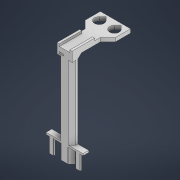
# Autodesk Inventor part: Vertical Beam Prototype
Saved by Autodesk Inventor 2022 (Build 260153000, 153)
## iProperties
Created: 2021-05-30
Part Number: Vertical Beam Prototype
Material: Generic
Document SubType Name: Modeling
Designer: sidsa
Density: 1 g/cm^3
Appearance: Default
Author: sidsa
## iProperties of the stored document Vertical Beam Prototype_3DPrint.ipt
Created: 2021-05-30
Part Number: Vertical Beam Prototype_3DPrint
Material: Generic
Document SubType Name: Modeling
Designer: sidsa
Density: 1 g/cm^3
Appearance: Default
Author: sidsa
Autodesk Inventor part; units mm, degrees
ref_plane "YZ Plane" through (0, 0, 0) normal (1, 0, 0) x (0, 1, 0)
ref_plane "XZ Plane" through (0, 0, 0) normal (0, 1, 0) x (-1, 0, 0)
ref_plane "XY Plane" through (0, 0, 0) normal (0, 0, 1) x (1, 0, 0)
sketch "Sketch1" plane through (0, 0, 0) normal (0, 0, 1) x (1, 0, 0)
  line L0 (0, 0) -> (25.4, 0)
  line L1 (25.4, 0) -> (25.4, 165.1)
  line L2 (25.4, 165.1) -> (0, 165.1)
  line L3 (0, 165.1) -> (0, 0)
  line L4 (16.2837, 38.7604) -> (19.9133, 32.4739)
  line L5 (19.9133, 32.4739) -> (16.2837, 26.1874)
  line L6 (16.2837, 26.1874) -> (9.0247, 26.1874)
  line L7 (9.0247, 26.1874) -> (5.3952, 32.4739)
  line L8 (5.3952, 32.4739) -> (9.0247, 38.7604)
  line L9 (9.0247, 38.7604) -> (16.2837, 38.7604)
  line L10 (12.7, 0) -> (12.6542, 32.4739)
  dimension "d0" = 25.4
  dimension "d1" = 165.1
  dimension "d2" = 12.573
  dimension "d3" = 26.1874
  constraints: 22 end point, 3 parallel, 1 horizontal, 1 midpoint, 1 perpendicular, 13 other
  measures "d0" distance of L1.end L2.end
  measures "d1" distance of L0.end L1.end
  measures "d2" distance between parallel lines of L6 L9
  measures "d3" distance between parallel lines of L0 L6
extrude "Extrusion1" add sketch "Sketch1" along normal blind 3.175
sketch "Sketch2" plane through (0, 0, 0) normal (0, 0, -1) x (-1, 0, 0)
  line L0 (-25.4, 0) -> (-25.4, 165.1) projected
  line L1 (0, 0) -> (-25.4, 0) projected
  line L2 (0, 165.1) -> (0, 0) projected
  line L3 (-25.4, 165.1) -> (0, 165.1) projected
  line L4 (-16.2837, 26.1874) -> (-9.0247, 26.1874) projected
  line L5 (-19.9133, 32.4739) -> (-16.2837, 26.1874) projected
  line L6 (-16.2837, 38.7604) -> (-19.9133, 32.4739) projected
  line L7 (-9.0247, 38.7604) -> (-16.2837, 38.7604) projected
  line L8 (-5.3952, 32.4739) -> (-9.0247, 38.7604) projected
  line L9 (-9.0247, 26.1874) -> (-5.3952, 32.4739) projected
  line L10 (-16.2984, 26.1967) -> (-19.9179, 32.4658) projected
  line L11 (-5.4399, 32.4658) -> (-9.0594, 26.1967) projected
  line L12 (-9.0594, 26.1967) -> (-16.2984, 26.1967) projected
  line L13 (-16.2984, 26.1967) -> (-19.9179, 32.4658) projected
  line L14 (-19.9179, 32.4658) -> (-16.2984, 38.735) projected
  line L15 (-16.2984, 38.735) -> (-9.0594, 38.735) projected
  line L16 (-9.0594, 38.735) -> (-5.4399, 32.4658) projected
  line L17 (-41.2539, 1.27) -> (-34.9039, 1.27) projected
  line L18 (15.8961, 1.27) -> (15.8961, 63.5) projected
  line L19 (-41.2539, 63.5) -> (15.8961, 63.5) projected
  line L20 (-41.2539, 1.27) -> (-41.2539, 63.5) projected
  line L21 (6.3711, 1.27) -> (6.3711, 26.67) projected
  line L22 (6.3711, 26.67) -> (9.5461, 26.67) projected
  line L23 (9.5461, 26.67) -> (9.5461, 1.27) projected
  line L24 (9.5461, 1.27) -> (15.8961, 1.27) projected
  line L25 (-34.9039, 1.27) -> (-34.9039, 26.67) projected
  line L26 (-34.9039, 26.67) -> (-31.7289, 26.67) projected
  line L27 (-31.7289, 26.67) -> (-31.7289, 1.27) projected
  line L28 (-31.7289, 1.27) -> (6.3711, 1.27) projected
  dimension "d32" = 12.573
  dimension "d33" = 12.5383
  measures "d32" distance between parallel lines of L7 L4
  measures "d33" distance between parallel lines of L12 L15
extrude "Extrusion2" add sketch "Sketch2" along normal blind 6.35 and the other way blind 3.175 contours L5 L12 L11 L16 L15 L6 L7 L8 L9 L4 | L5 L6 L15 L16 L11 L12
sketch "Sketch3" plane through (0, 0, 3.175) normal (0, 0, 1) x (1, 0, 0)
  line L0 (25.4, 0) -> (25.4, 165.1) projected
  line L1 (25.4, 165.1) -> (0, 165.1) projected
  line L2 (0, 165.1) -> (0, 0) projected
  line L3 (0, 0) -> (25.4, 0) projected
extrude "Extrusion3" add sketch "Sketch3" along normal blind 6.35
chamfer "Chamfer1" distance 6.35 angle 45 2 edges at (25.4, 82.55, 9.525) (0, 82.55, 9.525)
sketch "Sketch5" plane through (9.0247, 38.7604, 0) normal (0, 1, 0) x (1, 0, 0)
  line L0 (7.259, 0) -> (7.259, 6.35) projected
  line L1 (32.2292, 2.54) -> (-24.9208, 2.54) projected
  line L2 (0, 0) -> (0, 6.35) projected
  line L3 (7.259, 0) -> (7.259, 6.35) projected
  line L4 (0, 6.35) -> (0, 0) projected
  line L5 (7.259, 2.54) -> (0, 2.54)
  line L6 (0, 2.54) -> (0, 6.35)
  line L7 (0, 6.35) -> (7.259, 6.35)
  line L8 (7.259, 6.35) -> (7.259, 2.54)
  line L9 (5.989, 3.175) -> (1.27, 3.175)
  line L10 (1.27, 3.175) -> (1.27, 5.715)
  line L11 (1.27, 5.715) -> (5.989, 5.715)
  line L12 (5.989, 5.715) -> (5.989, 3.175)
  point P0 (-9.0247, 0)
  dimension "d25" = 0.635
  dimension "d26" = 1.27
  dimension "d27" = 0.635
  dimension "d28" = 1.27
  dimension "d29" = 2.54
  constraints: 16 end point, 4 parallel, 2 horizontal, 2 perpendicular, 2 point on line
  measures "d25" distance between parallel lines of L1 L9
  measures "d26" distance between parallel lines of L2 L10
  measures "d27" distance between parallel lines of L7 L11
  measures "d28" distance between parallel lines of L0 L12
  measures "d29" distance between parallel lines of L11 L9
extrude "Extrusion5" cut sketch "Sketch5" against normal blind 12.7 contours L9 L10 L11 L12
sketch "Sketch6" plane through (0, 0, 0) normal (0, 0, -1) x (-1, 0, 0)
  line L0 (-25.4, 0) -> (-25.4, 165.1) projected
  line L1 (0, 0) -> (-25.4, 0) projected
  line L2 (0, 165.1) -> (0, 0) projected
  line L3 (-25.4, 165.1) -> (0, 165.1) projected
  line L4 (-16.2837, 26.1874) -> (-9.0247, 26.1874) projected
  line L5 (-19.9133, 32.4739) -> (-16.2837, 26.1874) projected
  line L6 (-16.2837, 38.7604) -> (-19.9133, 32.4739) projected
  line L7 (-9.0247, 38.7604) -> (-16.2837, 38.7604) projected
  line L8 (-5.3952, 32.4739) -> (-9.0247, 38.7604) projected
  line L9 (-9.0247, 26.1874) -> (-5.3952, 32.4739) projected
  line L10 (0, 165.1) -> (0, 0) projected
  line L11 (-25.4, 165.1) -> (0, 165.1)
  line L12 (0, 165.1) -> (0, 158.75)
  line L13 (0, 158.75) -> (-25.4, 158.75)
  line L14 (-25.4, 158.75) -> (-25.4, 165.1)
  point P0 (-25.4, 158.75)
  dimension "d34" = 6.35
  constraints: 8 end point, 2 parallel, 1 horizontal, 1 perpendicular, 1 point on line
  measures "d34" distance of L11.end L12.end
extrude "Extrusion6" add sketch "Sketch6" along normal blind 76.2 contours L0 L3 L2 L13
sketch "Sketch7" plane through (0, 0, 3.175) normal (-1, 0, 0) x (0, 0, 1)
  line L0 (-79.375, 165.1) -> (0, 165.1) projected
  line L1 (-3.175, 158.75) -> (-79.375, 158.75) projected
  line L2 (-79.375, 165.1) -> (-53.975, 165.1)
  line L3 (-53.975, 165.1) -> (-53.975, 158.75)
  line L4 (-53.975, 158.75) -> (-79.375, 158.75)
  line L5 (-79.375, 158.75) -> (-79.375, 165.1)
  point P0 (-3.175, 0)
  dimension "d37" = 25.4
  constraints: 8 end point, 2 parallel, 1 horizontal, 1 perpendicular, 1 point on line
  measures "d37" distance of L3.end L4.end
extrude "Extrusion7" add sketch "Sketch7" along normal blind 12.7
sketch "Sketch8" plane through (25.4, 0, 3.175) normal (1, 0, 0) x (0, 0, -1)
  line L0 (79.375, 165.1) -> (0, 165.1) projected
  line L1 (79.375, 165.1) -> (53.975, 165.1)
  line L2 (53.975, 165.1) -> (53.975, 158.75)
  line L3 (53.975, 158.75) -> (79.375, 158.75)
  line L4 (79.375, 158.75) -> (79.375, 165.1)
  point P0 (3.175, 0)
  dimension "d40" = 25.4
  dimension "d41" = 6.35
  constraints: 8 end point, 2 parallel, 1 horizontal, 1 perpendicular
  measures "d40" distance of L3.end L2.end
  measures "d41" distance of L2.end L1.end
extrude "Extrusion8" add sketch "Sketch8" along normal blind 12.7
sketch "Sketch9" plane through (6.35, 165.1, 9.525) normal (0, 1, 0) x (1, 0, 0)
  circle A0 centre (-6.227, 72.0756) radius 6.55 projected
  circle A1 centre (19.373, 72.0756) radius 6.55 projected
  line L0 (31.75, 85.725) -> (31.75, 60.325) projected
  line L1 (-19.05, 60.325) -> (-19.05, 85.725) projected
  line L2 (31.75, 60.325) -> (31.75, 85.725) projected
  line L3 (31.75, 71.286) -> (25.8752, 71.286)
  line L4 (12.8707, 71.286) -> (-19.05, 71.286)
  line L5 (31.75, 71.286) -> (27.2796, 71.286)
  line L6 (27.2796, 71.286) -> (19.1516, 71.286)
  circle A2 centre (19.1516, 71.286) radius 8.128
  line L7 (-19.05, 71.286) -> (-6.4516, 71.286)
  circle A3 centre (-6.4516, 71.286) radius 8.128
  point P0 (-6.35, 9.525)
  point P1 (1.6764, 71.286)
  point P2 (-14.5796, 71.286)
  point P3 (-12.7293, 71.286)
  point P4 (0.2752, 71.286)
  dimension "d49" = 25.6
  dimension "d50" = 4.4704
  dimension "d51" = 8.128
  dimension "d52" = 16.256
  dimension "d53" = 12.5984
  dimension "d54" = 16.256
  constraints: 10 end point, 5 point on line, 2 centre point, 2 coincident, 2 perpendicular, 2 point on circle
  measures "d49" distance of A0.centre A1.centre
  measures "d50" distance of L3.start L5.end
  measures "d51" distance of L5.end L6.end
  measures "d52" diameter of A2
  measures "d53" distance of L4.end L7.end
  measures "d54" diameter of A3
extrude "Extrusion9" cut sketch "Sketch9" against normal blind 6.35
chamfer "Chamfer5" distance 12.7 angle 45 2 edges at (25.4, 161.925, -50.8) (0, 161.925, -50.8)
chamfer "Chamfer6" distance 6.35 angle 45 1 edges at (12.7, 158.75, 0)
sketch "Sketch10" plane through (0, 0, 3.175) normal (-1, 0, 0) x (0, 0, 1)
  line L0 (-41.275, 158.75) -> (-41.275, 165.1) projected
  line L1 (-9.525, 158.75) -> (-41.275, 158.75) projected
  line L2 (-3.175, 152.4) -> (-9.525, 158.75) projected
  line L3 (-3.175, 152.4) -> (-3.175, 0) projected
  line L4 (-3.175, 0) -> (0, 0) projected
  line L5 (0, 165.1) -> (0, 0) projected
  line L6 (-41.275, 165.1) -> (0, 165.1) projected
  line L7 (-9.525, 158.75) -> (-9.525, 165.1)
  line L8 (-3.175, 152.4) -> (6.35, 152.4)
  line L9 (6.35, 0) -> (6.35, 165.1) projected
  line L10 (6.35, 165.1) -> (-9.525, 165.1)
  constraints: 6 end point, 2 perpendicular, 2 point on line, 1 parallel
extrude "Extrusion10" add sketch "Sketch10" against normal blind 25.4 contours L7 L6 L5 L8 L2 | L10 L9 L8 L5
sketch "Sketch11" plane through (0, 0, 9.525) normal (0, 0, 1) x (1, 0, 0)
  line L0 (3.81, 157.48) -> (11.43, 157.48)
  line L1 (11.43, 157.48) -> (11.43, 154.94)
  line L2 (11.43, 154.94) -> (3.81, 154.94)
  line L3 (3.81, 154.94) -> (3.81, 157.48)
  line L4 (0, 152.4) -> (0, 165.1) projected
  line L5 (0, 165.1) -> (25.4, 165.1) projected
  point P0 (0, 0)
  dimension "d65" = 2.54
  dimension "d66" = 7.62
  dimension "d67" = 3.81
  dimension "d68" = 7.62
  constraints: 8 end point, 2 parallel, 1 horizontal, 1 perpendicular
  measures "d65" distance of L2.end L0.start
  measures "d66" distance of L1.end L2.end
  measures "d67" distance between parallel lines of L4 L3
  measures "d68" distance between parallel lines of L5 L0
extrude "Extrusion11" cut sketch "Sketch11" against normal blind 25.4
chamfer "Chamfer7" distance 0.7937 angle 45 4 edges at (7.62, 157.48, -5.08) (11.43, 156.21, -3.81) (3.81, 156.21, -3.81) (7.62, 154.94, -2.54)
sketch "Sketch12" plane through (0, 0, 0) normal (0, -1, 0) x (1, 0, 0)
  line L0 (0, 3.175) -> (6.35, 9.525) projected
  line L1 (0, 0) -> (0, 3.175) projected
  line L2 (0, 0) -> (25.4, 0) projected
  line L3 (25.4, 0) -> (25.4, 3.175) projected
  line L4 (19.05, 9.525) -> (25.4, 3.175) projected
  line L5 (6.35, 9.525) -> (19.05, 9.525) projected
  line L6 (6.35, 9.525) -> (19.05, 9.525) projected
  line L7 (12.7, 9.525) -> (-18.415, 9.525)
  line L8 (12.7, 9.525) -> (43.815, 9.525)
  line L9 (43.815, 9.525) -> (43.815, 0)
  line L10 (43.815, 0) -> (-18.415, 0)
  line L11 (-18.415, 0) -> (-18.415, 9.525)
  dimension "d74" = 31.115
  dimension "d75" = 31.115
  constraints: 10 end point, 3 perpendicular, 2 point on line, 1 midpoint
  measures "d74" distance of L7.start L7.end
  measures "d75" distance of L7.start L8.end
extrude "Extrusion12" add sketch "Sketch12" against normal blind 3.175 contours L1 L10 L11 L7 L0 | L3 L4 L8 L9 L10
sketch "Sketch13" plane through (0, 3.175, 0) normal (0, 1, 0) x (1, 0, 0)
  line L0 (0, 0) -> (-18.415, 0) projected
  line L1 (-18.415, 0) -> (-18.415, -9.525) projected
  line L2 (-18.415, -9.525) -> (6.35, -9.525) projected
  line L3 (0, -3.175) -> (6.35, -9.525) projected
  line L4 (0, 0) -> (0, -3.175) projected
  line L5 (19.05, -9.525) -> (43.815, -9.525) projected
  line L6 (43.815, -9.525) -> (43.815, 0) projected
  line L7 (43.815, 0) -> (25.4, 0) projected
  line L8 (25.4, -3.175) -> (25.4, 0) projected
  line L9 (19.05, -9.525) -> (25.4, -3.175) projected
  line L10 (0, -9.525) -> (25.4, -9.525) projected
  line L11 (12.7, -9.525) -> (12.7, 5.0983)
  line L12 (9.0247, 6.35) -> (16.2837, 6.35) projected
  line L13 (43.815, -9.525) -> (-18.415, -9.525) projected
  line L14 (-13.335, -9.525) -> (-5.842, -9.525)
  line L15 (-5.842, -9.525) -> (-5.842, -6.35)
  line L16 (-5.842, -6.35) -> (-13.335, -6.35)
  line L17 (-13.335, -6.35) -> (-13.335, -9.525)
  line L18 (38.735, -9.525) -> (31.242, -9.525)
  line L19 (31.242, -9.525) -> (31.242, -6.35)
  line L20 (31.242, -6.35) -> (38.735, -6.35)
  line L21 (38.735, -6.35) -> (38.735, -9.525)
  point P0 (31.242, -9.525)
  dimension "d85" = 3.175
  dimension "d86" = 5.08
  dimension "d87" = 12.573
  constraints: 18 end point, 4 symmetric about line, 2 parallel, 2 perpendicular, 1 horizontal, 1 midpoint, 1 point on line
  measures "d85" distance between parallel lines of L13 L16
  measures "d86" distance between parallel lines of L1 L17
  measures "d87" distance between parallel lines of L1 L15
extrude "Extrusion13" add sketch "Sketch13" along normal blind 25.4 contours L17 L16 L15 L2 | L19 L20 L21 L5
fillet "Fillet1" radius 3.175 2 edges at (43.815, 1.5875, 9.525) (-18.415, 1.5875, 9.525)
sketch "Sketch14" plane through (0, 28.575, 0) normal (0, 1, 0) x (1, 0, 0)
  point P0 (0, 0)
sketch "Sketch15" plane through (0, 28.575, 0) normal (0, 1, 0) x (1, 0, 0)
  line L0 (0, 0) -> (-18.415, 0)
  line L1 (-18.415, 0) -> (-18.415, -9.525)
  line L2 (-18.415, -9.525) -> (6.35, -9.525)
  line L3 (0, -3.175) -> (6.35, -9.525)
  line L4 (0, 0) -> (0, -3.175)
  line L5 (19.05, -9.525) -> (43.815, -9.525)
  line L6 (43.815, -9.525) -> (43.815, 0)
  line L7 (43.815, 0) -> (25.4, 0)
  line L8 (25.4, -3.175) -> (25.4, 0)
  line L9 (19.05, -9.525) -> (25.4, -3.175)
  line L10 (0, -9.525) -> (25.4, -9.525)
  line L11 (12.7, -9.525) -> (12.7, 5.0983)
  line L12 (9.0247, 6.35) -> (16.2837, 6.35)
  line L13 (43.815, -9.525) -> (-18.415, -9.525)
  line L14 (-13.335, -9.525) -> (-5.715, -9.525)
  line L15 (-5.715, -9.525) -> (-5.715, -6.35)
  line L16 (-5.715, -6.35) -> (-13.335, -6.35)
  line L17 (-13.335, -6.35) -> (-13.335, -9.525)
  line L18 (38.735, -9.525) -> (31.115, -9.525)
  line L19 (31.115, -6.35) -> (38.735, -6.35)
  line L20 (38.735, -6.35) -> (38.735, -9.525)
  line L21 (31.115, -9.525) -> (31.115, -6.35)
  dimension "d91" = 3.175
  dimension "d92" = 5.08
  dimension "d93" = 12.7
  constraints: 44 end point, 4 symmetric about line, 2 parallel, 2 perpendicular, 1 horizontal, 1 midpoint, 1 point on line
  measures "d91" distance between parallel lines of L13 L16
  measures "d92" distance between parallel lines of L1 L17
  measures "d93" distance between parallel lines of L1 L15
extrude "Extrusion14" add sketch "Sketch15" against normal blind 3.175 contours L4 L3 L2 L15 L16 L17 L1 L0 | L9 L8 L7 L6 L5 L20 L19 L21
sketch "Sketch16" plane through (0, 3.175, 0) normal (0, 1, 0) x (1, 0, 0)
  arc A0 (-18.415, -6.35) -> (-15.24, -9.525) centre (-15.24, -6.35) ccw projected
  line L0 (-15.24, -9.525) -> (-13.335, -9.525) projected
  line L1 (-13.335, -9.525) -> (-13.335, -6.35) projected
  line L2 (-13.335, -6.35) -> (-5.842, -6.35) projected
  line L3 (-5.842, -6.35) -> (-5.842, -9.525) projected
  line L4 (-5.842, -9.525) -> (6.35, -9.525) projected
  line L5 (0, -3.175) -> (6.35, -9.525) projected
  line L6 (0, 0) -> (0, -3.175) projected
  line L7 (0, 0) -> (-18.415, 0) projected
  line L8 (-18.415, 0) -> (-18.415, -6.35) projected
  arc A1 (40.64, -9.525) -> (43.815, -6.35) centre (40.64, -6.35) ccw projected
  line L9 (43.815, -6.35) -> (43.815, 0) projected
  line L10 (43.815, 0) -> (25.4, 0) projected
  line L11 (25.4, -3.175) -> (25.4, 0) projected
  line L12 (19.05, -9.525) -> (25.4, -3.175) projected
  line L13 (19.05, -9.525) -> (31.242, -9.525) projected
  line L14 (31.242, -9.525) -> (31.242, -6.35) projected
  line L15 (31.242, -6.35) -> (38.735, -6.35) projected
  line L16 (38.735, -6.35) -> (38.735, -9.525) projected
  line L17 (38.735, -9.525) -> (40.64, -9.525) projected
extrude "Extrusion15" cut sketch "Sketch16" against normal blind 3.175
chamfer "Chamfer11" distance 0.635 angle 45 8 edges at (31.242, 12.7, 6.35) (31.242, 14.2875, 9.525) (38.735, 12.7, 9.525) (38.735, 12.7, 6.35) (-5.842, 12.7, 6.35) (-13.335, 12.7, 6.35) (-13.335, 12.7, 9.525) (-5.842, 14.2875, 9.525)
chamfer "Chamfer12" distance 0.635 angle 45 4 edges at (6.35, 12.7, 9.525) (0, 12.7, 3.175) (19.05, 12.7, 9.525) (25.4, 12.7, 3.175)
chamfer "Chamfer13" distance 0.635 angle 45 26 edges at (25.1755, 0, 3.082) (31.242, 0, 7.9375) (3.175, 0, 6.35) (12.7, 0, 0) (0, 0, 1.27) (0.2245, 0, 3.082) (12.7, 0, 9.525) (6.443, 0, 9.3005) (18.957, 0, 9.3005) (38.4175, 0, 6.6675) (34.9885, 0, 6.35) (22.225, 0, 6.35) (38.735, 0, 7.9375) (38.4175, 0, 9.2075) (34.9885, 0, 9.525) (31.5595, 0, 9.2075) (31.5595, 0, 6.6675) (25.4, 0, 1.27) (-13.335, 0, 7.9375) (-6.1595, 0, 6.6675) (-13.0175, 0, 9.2075) (-13.0175, 0, 6.6675) (-9.5885, 0, 9.525) (-9.5885, 0, 6.35) (-6.1595, 0, 9.2075) (-5.842, 0, 7.9375)
sketch "Sketch18" plane through (0, 0, 9.525) normal (0, 0, 1) x (1, 0, 0)
  line L0 (18.415, 0.635) -> (6.985, 0.635) projected
  line L1 (18.415, 25.4) -> (18.415, 0.635) projected
  line L2 (31.115, 25.4) -> (18.415, 25.4) projected
  line L3 (31.115, 28.575) -> (31.115, 25.4) projected
  line L4 (19.05, 28.575) -> (31.115, 28.575) projected
  line L5 (19.05, 152.4) -> (19.05, 28.575) projected
  line L6 (19.05, 152.4) -> (25.4, 152.4) projected
  line L7 (25.4, 165.1) -> (25.4, 152.4) projected
  line L8 (0, 165.1) -> (25.4, 165.1) projected
  line L9 (0, 152.4) -> (0, 165.1) projected
  line L10 (0, 152.4) -> (6.35, 152.4) projected
  line L11 (6.35, 28.575) -> (6.35, 152.4) projected
  line L12 (-5.715, 28.575) -> (6.35, 28.575) projected
  line L13 (-5.715, 28.575) -> (-5.715, 25.4) projected
  line L14 (6.985, 25.4) -> (-5.715, 25.4) projected
  line L15 (6.985, 0.635) -> (6.985, 25.4) projected
  line L16 (11.43, 157.48) -> (11.43, 154.94) projected
  line L17 (11.43, 154.94) -> (3.81, 154.94) projected
  line L18 (3.81, 154.94) -> (3.81, 157.48) projected
  line L19 (3.81, 157.48) -> (11.43, 157.48) projected
  line L20 (0, 152.4) -> (0, 165.1) projected
  line L21 (0, 165.1) -> (3.81, 165.1)
  line L22 (3.81, 165.1) -> (3.81, 168.91)
  line L23 (3.81, 168.91) -> (0, 168.91)
  line L24 (0, 168.91) -> (0, 165.1)
  line L25 (0, 165.1) -> (25.4, 165.1) projected
  line L26 (25.4, 165.1) -> (21.59, 165.1)
  line L27 (21.59, 165.1) -> (21.59, 168.91)
  line L28 (21.59, 168.91) -> (25.4, 168.91)
  line L29 (25.4, 168.91) -> (25.4, 165.1)
  point P0 (0, 0)
  dimension "d118" = 3.81
  dimension "d119" = 3.81
  dimension "d120" = 3.81
  constraints: 16 end point, 4 parallel, 2 horizontal, 2 perpendicular, 1 collinear
  measures "d118" distance of L21.end L22.end
  measures "d119" distance of L22.end L23.end
  measures "d120" distance of L27.end L28.end
extrude "Extrusion16" add sketch "Sketch18" against normal blind 38.1 contours L8 L27 L28 L29 | L24 L23 L22 L8
sketch "Sketch19" plane through (-12.7, 165.1, -76.2) normal (0, 1, 0) x (1, 0, 0)
  line L0 (34.29, -47.625) -> (38.1, -47.625) projected
  line L1 (38.1, -38.1) -> (38.1, -47.625) projected
  line L2 (50.8, -25.4) -> (38.1, -38.1) projected
  line L3 (50.8, 0) -> (50.8, -25.4) projected
  line L4 (50.8, 0) -> (0, 0) projected
  line L5 (0, -25.4) -> (0, 0) projected
  line L6 (12.7, -38.1) -> (0, -25.4) projected
  line L7 (12.7, -38.1) -> (12.7, -47.625) projected
  line L8 (12.7, -47.625) -> (16.51, -47.625) projected
  line L9 (16.51, -47.625) -> (16.51, -85.725) projected
  line L10 (16.51, -85.725) -> (34.29, -85.725) projected
  line L11 (34.29, -85.725) -> (34.29, -47.625) projected
  circle A0 centre (12.5984, -14.439) radius 8.128 projected
  circle A1 centre (38.2016, -14.439) radius 8.128 projected
  line L12 (1.1071, -14.4356) -> (12.6018, -25.9303)
  line L13 (12.6018, -25.9303) -> (24.0897, -14.4423)
  line L14 (24.0897, -14.4423) -> (12.595, -2.9476)
  line L15 (12.595, -2.9476) -> (1.1071, -14.4356)
  line L16 (1.1071, -14.4356) -> (24.0897, -14.4423) construction
  line L17 (12.6018, -25.9303) -> (12.595, -2.9476) construction
  circle A2 centre (12.5984, -14.439) radius 8.128 projected
  line L18 (4.4694, -17.7979) -> (4.4714, -11.0712)
  line L19 (50.8, 0) -> (0, 0) projected
  line L20 (25.4, 0) -> (25.4, -35.2188)
  line L21 (20.7294, -17.8027) -> (20.7234, -11.0665)
  line L22 (38.1982, -25.9303) -> (26.7103, -14.4423)
  line L23 (26.7103, -14.4423) -> (38.205, -2.9476)
  line L24 (38.205, -2.9476) -> (49.6929, -14.4356)
  line L25 (46.3341, -29.8659) -> (46.3254, 0)
  line L26 (49.6929, -14.4356) -> (38.1982, -25.9303)
  line L27 (30.0706, -17.8027) -> (30.0863, 0)
  point P0 (12.7, -76.2)
  point P1 (20.7294, -17.7932)
  point P2 (46.3306, -17.7979)
  point P3 (46.3286, -11.0712)
  point P4 (30.0706, -17.7932)
  point P5 (30.0766, -11.0665)
  point P6 (32.6547, -8.4979)
  point P7 (43.949, -8.6916)
  point P8 (6.851, -8.6916)
  point P9 (18.1453, -8.4979)
  constraints: 30 end point, 13 point on line, 10 symmetric about line, 3 midpoint, 3 perpendicular, 2 parallel
extrude "Extrusion17" cut sketch "Sketch19" against normal blind 25.4 contours A1 L23 L24 | A0 L15 L14
sketch "Sketch20" plane through (-12.7, 165.1, -76.2) normal (0, 1, 0) x (1, 0, 0)
  point P0 (12.7, -76.2)
sketch "Sketch21" plane through (0, 0, 9.525) normal (0, 0, 1) x (1, 0, 0)
  line L0 (-18.415, 28.575) -> (-18.415, 25.4) projected
  line L1 (43.815, 28.575) -> (43.815, 25.4) projected
  line L2 (-18.415, 28.575) -> (43.815, 28.575)
  line L3 (43.815, 28.575) -> (43.815, 25.4)
  line L4 (43.815, 25.4) -> (-18.415, 25.4)
  line L5 (-18.415, 25.4) -> (-18.415, 28.575)
  point P0 (0, 0)
  constraints: 8 end point, 2 parallel, 1 horizontal, 1 perpendicular
extrude "Extrusion18" add sketch "Sketch21" against normal blind 5.08
body "Solid1"
